spatula (Autodesk Fusion 360 design; units mm, degrees)
Autodesk Fusion 360 part; units mm, degrees
note: some values were not read from the file. Set by a fixed rule: which sketch regions a step uses.
sketch "Sketch1" plane through (0, 0, 0) normal (0, 1, 0) x (1, 0, 0)
  line L0 (0, 0) -> (-15, 0)
  line L1 (-15, 0) -> (-15, -4)
  line L2 (-15, -4) -> (0, -4)
  line L3 (0, -4) -> (0, 0)
  dimension "d1" = 4
  dimension "d2" = 15
  constraint horizontal L0
  constraint vertical L1
  constraint horizontal L2
  constraint vertical L3
  constraint coincident L0.start L3.end
  measures "d1" distance of L0.start L2.end
  measures "d2" distance of L1.end L2.end
extrude "Extrude1" add sketch "Sketch1" along normal blind 50
sketch "Sketch2" plane through (0, 50, 0) normal (0, 1, 0) x (-1, 0, 0)
  line L0 (0, 4) -> (0, 0)
  line L1 (0, 0) -> (15, 0)
  line L2 (15, 0) -> (15, 4)
  line L3 (15, 4) -> (0, 4)
  line L4 (-3.5, 0) -> (18.5, 0)
  line L5 (18.5, 0) -> (18.5, 7.5)
  line L6 (18.5, 7.5) -> (-3.5, 7.5)
  line L7 (-3.5, 7.5) -> (-3.5, 0)
  dimension "d5" = 3.5
  dimension "d6" = 3.5
  dimension "d7" = 3.5
  constraint horizontal L4
  constraint vertical L5
  constraint horizontal L6
  constraint vertical L7
  constraint collinear L1 L4
  measures "d5" distance of L2 L5
  measures "d6" distance of L0 L7
  measures "d7" distance of L3 L6
ref_plane "WorkPlane1" through (-7.5, 210, 2) normal (0, 1, 0) x (-1, 0, 0)
sketch "Sketch3" plane through (0, 210, 0) normal (0, 1, 0) x (1, 0, 0)
  line L0 (8, 0) -> (-22, 0)
  line L1 (-22, 0) -> (-22, -10)
  line L2 (-22, -10) -> (8, -10)
  line L3 (8, -10) -> (8, 0)
  dimension "d9" = 22
  dimension "d10" = 8
  dimension "d11" = 10
  constraint horizontal L0
  constraint vertical L1
  constraint horizontal L2
  constraint vertical L3
  constraint coincident origin L0
  measures "d9" distance of origin L1
  measures "d10" distance of origin L3
  measures "d11" distance of L0.end L1.end
loft "Loft1" add profiles "Sketch2", "Sketch3" section 1 section 2
fillet "Fillet1" radius 3 8 edges at (5.75, 130, 8.75) (-7, 210, 10) (-20.25, 130, 8.75) (-22, 210, 5) (8, 210, 5) (-18.5, 50, 3.75) (-7.5, 50, 7.5) (3.5, 50, 3.75)
fillet "Fillet2" radius 1 9 edges at (-15.2825, 50, 0) (-17.6629, 50.8556, 0) (-20.2486, 129.9344, 0) (-21.078, 209.098, 0) (-7.0096, 210, 0) (7.0654, 209.0913, 0) (5.7476, 129.9157, 0) (2.6745, 50.8491, 0) (0.2916, 50, 0)
sketch "Sketch4" plane through (0, 0, 4) normal (0, 0, 1) x (-1, 0, 0)
  line L0 (15, 0) -> (0, 0)
  line L1 (0, 0) -> (0, -50)
  line L2 (0, -50) -> (15, -50)
  line L3 (15, -50) -> (15, 0)
  line L4 (7.5, 0) -> (7.5, -50)
  circle A0 centre (0, -25) radius 1
  line L5 (7.5, -25) -> (0, -25)
  line L6 (0, -6) -> (-1.3, -10)
  line L7 (-1.3, -10) -> (0, -10)
  line L8 (0, -35) -> (-1.3, -39)
  line L9 (-1.3, -39) -> (0, -39)
  line L10 (15, -6) -> (16.3, -10)
  line L11 (16.3, -10) -> (15, -10)
  circle A1 centre (15, -25) radius 1
  line L12 (15, -35) -> (16.3, -39)
  line L13 (16.3, -39) -> (15, -39)
  dimension "d16" = 2
  dimension "d17" = 6
  dimension "d18" = 1.3
  dimension "d19" = 4
  dimension "d20" = 4
  dimension "d21" = 10
  dimension "d22" = 1.3
  constraint midpoint L0 L4.start
  constraint midpoint L2 L4.end
  constraint coincident L1 A0.centre
  constraint midpoint L4 L5.start
  constraint midpoint L1 A0.centre
  constraint coincident A0.centre L5.end
  constraint coincident L1 L6.start
  constraint coincident L1 L7.end
  constraint perpendicular L1 L7
  constraint coincident L1 L8.start
  constraint coincident L1 L9.end
  constraint perpendicular L1 L9
  constraint symmetric L4 A0 A1
  constraint symmetric L4 L6.start L10.start
  constraint symmetric L4 L6.end L10.end
  constraint symmetric L4 L7.end L11.end
  constraint symmetric L4 L8.start L12.start
  constraint symmetric L4 L8.end L12.end
  constraint symmetric L4 L9.end L13.end
  measures "d16" diameter of A0
  measures "d17" distance of L0.end L6.start
  measures "d18" distance of L6.end L7.end
  measures "d19" distance of L6.start L7.end
  measures "d20" distance of L8.start L9.end
  measures "d21" distance of A0.centre L8.start
  measures "d22" distance of L8.end L9.end
extrude "Extrude2" add sketch "Sketch4" against normal blind 4 contours L3 L10 L11 | L1 L6 L7 | L3 A1 | L1 A0 | L1 L8 L9 | L3 L12 L13 picked at (15.3299, -25.0474)
equation "d6 = d5"
equation "d7 = d5"
equation "d20 = d19"
equation "d22 = d18"
